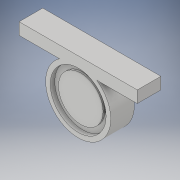
# Autodesk Inventor part: basicMount
Saved by Autodesk Inventor 2019.3 (Build 233278000, 278)
## iProperties
Created: 2019-01-13
Part Number: basicMount
Material: Generic
Document SubType Name: Modeling
Designer: steele
Density: 1 g/cm^3
Appearance: Default
Author: steele
Autodesk Inventor part; units mm, degrees
ref_plane "YZ Plane" through (0, 0, 0) normal (1, 0, 0) x (0, 1, 0)
ref_plane "XZ Plane" through (0, 0, 0) normal (0, 1, 0) x (-1, 0, 0)
ref_plane "XY Plane" through (0, 0, 0) normal (0, 0, 1) x (1, 0, 0)
sketch "Sketch1" plane through (0, 0, 0) normal (0, 0, 1) x (1, 0, 0)
  line L0 (63.5, -6.35) -> (63.5, 6.35)
  line L1 (63.5, 6.35) -> (-63.5, 6.35)
  line L2 (-63.5, 6.35) -> (-63.5, -6.35)
  line L3 (0, 0) -> (0, -35) construction
  line L4 (-63.5, -6.35) -> (-20.1042, -6.35)
  line L5 (20.1042, -6.35) -> (63.5, -6.35)
  line L6 (-63.5, -6.35) -> (-6.9307, -0.6931) construction
  line L7 (0, 0) -> (63.5, 6.35) construction
  line L8 (63.5, -6.35) -> (6.9307, -0.6931) construction
  line L9 (0, 0) -> (-63.5, 6.35) construction
  arc A0 (-20.1042, -6.35) -> (20.1042, -6.35) centre (0, -35) ccw
  dimension "d0" = 127
  dimension "d1" = 12.7
  dimension "d2" = 35
  constraints: 20 end point, 3 parallel, 2 horizontal, 2 perpendicular, 2 point on circle, 1 centre point, 1 coincident, 1 point on line, 1 vertical
  measures "d0" distance of L2.end L0.start
  measures "d1" distance of L0.end L0.start
  measures "d2" distance of L3.start L3.end
extrude "Extrusion1" add sketch "Sketch1" against normal blind 25.4
sketch "Sketch2" plane through (0, 0, 0) normal (0, 0, 1) x (1, 0, 0)
  arc A0 (-20.1042, -6.35) -> (20.1042, -6.35) centre (0, -35) ccw projected
  circle A1 centre (0, -35) radius 30
  point P0 (0, 0)
  dimension "d6" = 60
  constraints: 1 centre point, 1 coincident
  measures "d6" diameter of A1
extrude "Extrusion2" cut sketch "Sketch2" against normal blind 2.794
sketch "Sketch3" plane through (0, -35, -2.794) normal (0, 0, 1) x (1, 0, 0)
  circle A0 centre (0, 0) radius 30 projected
  circle A1 centre (0, 0) radius 31
  circle A2 centre (0, 0) radius 24
  point P0 (0, 35)
  dimension "d9" = 62
  dimension "d10" = 48
  constraints: 2 centre point, 2 coincident
  measures "d9" diameter of A1
  measures "d10" diameter of A2
extrude "Extrusion3" cut sketch "Sketch3" against normal blind 2 contours A0
sketch "Sketch4" plane through (0, -35, -4.794) normal (0, 0, 1) x (1, 0, 0)
  circle A0 centre (0, 0) radius 30 construction
  line L0 (0, 0) -> (34.925, 0) construction
  circle A1 centre (26.9875, 0) radius 3.0125
  point P0 (0, 35)
  constraints: 2 end point, 1 centre point, 1 horizontal, 1 point on line
extrude "Extrusion4" cut sketch "Sketch4" against normal through all
body "Solid1"
